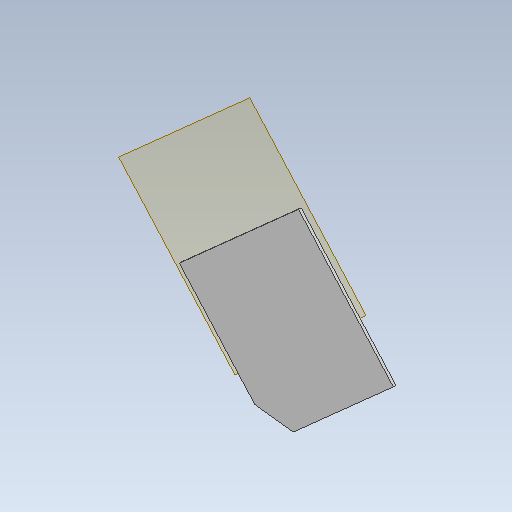
# Autodesk Inventor part: base_plate
Saved by Autodesk Inventor 2020.1 (Build 241239000, 239)
## iProperties
Created: 2019-07-16
Part Number: base_plate
Material: Générique
Document SubType Name: Modeling
Designer: Thibault
Density: 1 g/cm^3
Appearance: Par défaut
Author: Thibault
Autodesk Inventor part; units mm, degrees
ref_plane "YZ Plane" through (0, 0, 0) normal (1, 0, 0) x (0, 1, 0)
ref_plane "XZ Plane" through (0, 0, 0) normal (0, 1, 0) x (-1, 0, 0)
ref_plane "XY Plane" through (0, 0, 0) normal (0, 0, 1) x (1, 0, 0)
sketch "Anchor (screw side)" plane through (0, 0, 0) normal (0, 0, 1) x (1, 0, 0)
  circle A0 centre (93.7814, 50.2592) radius 1
  line L0 (91.2814, 51.2592) -> (88.2814, 51.2592)
  line L1 (88.2814, 51.2592) -> (88.2814, 49.2592)
  line L2 (88.2814, 49.2592) -> (91.2814, 49.2592)
  line L3 (91.2814, 49.2592) -> (91.2814, 51.2592)
  line L4 (99.2814, 51.2592) -> (96.2814, 51.2592)
  line L5 (96.2814, 51.2592) -> (96.2814, 49.2592)
  line L6 (96.2814, 49.2592) -> (99.2814, 49.2592)
  line L7 (99.2814, 49.2592) -> (99.2814, 51.2592)
  line L8 (91.2814, 51.2592) -> (96.2814, 49.2592) construction
  line L9 (96.2814, 51.2592) -> (91.2814, 49.2592) construction
  line L10 (86.2814, 53.2592) -> (101.2814, 53.2592) construction
  line L11 (101.2814, 53.2592) -> (101.2814, 47.2592) construction
  line L12 (101.2814, 47.2592) -> (86.2814, 47.2592) construction
  line L13 (86.2814, 47.2592) -> (86.2814, 53.2592) construction
  point P0 (103.5798, 50.1132)
  dimension "d27" = 2
  dimension "d28" = 3
  dimension "d29" = 2
  dimension "d30" = 3
  dimension "d32" = 5
  dimension "d34" = 2
  dimension "d35" = 2
  dimension "d36" = 2
  dimension "d37" = 2
  measures "d27" diameter of A0
  measures "d28" distance of L2.end L1.end
  measures "d29" distance of L1.end L0.end
  measures "d30" distance of L6.end L5.end
  measures "d32" distance between parallel lines of L5 L3
  measures "d34" distance between parallel lines of L0 L10
  measures "d35" distance between parallel lines of L12 L2
  measures "d36" distance between parallel lines of L11 L7
  measures "d37" distance between parallel lines of L13 L1
sketch "Anchor (nut side)" plane through (0, 0, 0) normal (0, 0, 1) x (1, 0, 0)
  line L0 (10, 0) -> (8.5, 0)
  line L1 (8.5, 0) -> (8.5, -2)
  line L2 (8.5, -2) -> (9.3, -2)
  line L3 (9.3, -2) -> (9.3, -4)
  line L4 (5.7, -4) -> (5.7, -2)
  line L5 (5.7, -2) -> (6.5, -2)
  line L6 (6.5, -2) -> (6.5, 0)
  line L7 (6.5, 0) -> (5, 0)
  line L8 (2, 0) -> (2, 2)
  line L9 (2, 0) -> (3, 0) construction
  line L10 (2, 2) -> (5, 2)
  line L11 (5, 2) -> (5, 0)
  line L12 (5, 2) -> (7, 2) construction
  line L13 (10, 0) -> (10, 2)
  line L14 (10, 2) -> (13, 2)
  line L15 (13, 2) -> (13, 0)
  line L16 (0, 0) -> (2, 0)
  line L17 (13, 0) -> (15, 0)
  line L18 (5.7, -4) -> (6.5, -4)
  line L19 (9.3, -4) -> (8.5, -4)
  line L20 (6.5, -4) -> (6.5, -6.25)
  line L21 (8.5, -4) -> (8.5, -6.25)
  line L22 (6.75, -6.5) -> (7.5, -6.5)
  arc A0 (6.5, -6.25) -> (6.75, -6.5) centre (6.75, -6.25) ccw
  arc A1 (8.25, -6.5) -> (8.5, -6.25) centre (8.25, -6.25) ccw
  line L23 (7.5, -7.2938) -> (7.5, -4.9797)
  line L24 (7.5, -6.5) -> (8.25, -6.5)
  point P0 (9.1321, -0.6227)
  point P1 (6.5, -6.5)
  point P2 (8.5, -6.5)
  dimension "d3" = 2
  dimension "d7" = 5
  dimension "d10" = 1.5
  dimension "d11" = 2
  dimension "d12" = 0.8
  dimension "d13" = 2
  dimension "d14" = 0.8
  dimension "d15" = 2
  dimension "d18" = 2
  dimension "d19" = 0.8
  dimension "d20" = 0.8
  dimension "d21" = 2.5
  dimension "d22" = 2.5
  dimension "d23" = 2
  dimension "d38" = 2
  dimension "d39" = 0.25
  dimension "d118" = 2
  dimension "d120" = 3
  measures "d3" distance of L16.start L8.start
  measures "d7" distance of L7.end L0.start
  measures "d10" distance of L0.start L0.end
  measures "d11" distance of L0.end L1.end
  measures "d12" distance of L1.end L2.end
  measures "d13" distance of L2.end L3.end
  measures "d14" distance of L4.end L5.end
  measures "d15" distance of L6.end L0.end
  measures "d18" distance of L15.end L17.end
  measures "d19" distance of L4.start L18.end
  measures "d20" distance of L3.end L19.end
  measures "d21" distance of L18.end point (6.5, -6.5)
  measures "d22" distance of L19.end point (8.5, -6.5)
  measures "d23" distance of L18.end L19.end
  measures "d38" distance between parallel lines of L16 L10
  measures "d39" radius of A0
  measures "d118" distance between parallel lines of L0 L14
  measures "d120" distance of L8.end L10.end
ref_plane "Plan de construction1" through (57.5253, 159.7091, 0) normal (0, 0, 1) x (-0.7464987, -0.6653869, 0)
sketch "Esquisse1" plane through (57.5253, 159.7091, 0) normal (0, 0, 1) x (-0.7464987, -0.6653869, 0)
  line L0 (0, 110) -> (103.4714, 110) projected
  line L1 (123.2302, 87.5455) -> (123.2302, 2) projected
  line L2 (0, 0) -> (123.2302, 0) projected
  line L3 (0, 108) -> (0, 2) projected
  line L4 (123.2302, 2) -> (123.2302, 0)
  line L5 (0, 2) -> (0, 0)
  line L6 (0, 108) -> (0, 110)
  line L7 (103.4714, 110) -> (123.2302, 87.5455)
  constraints: 8 end point, 2 equal length, 1 perpendicular
derived "shared_parameters.ipt"
extrude "Extrusion1" add sketch "Esquisse1" along normal blind 2
equation "\"d1\" = sheet_thickness"
equation "\"sheet_thickness\" = 2"
